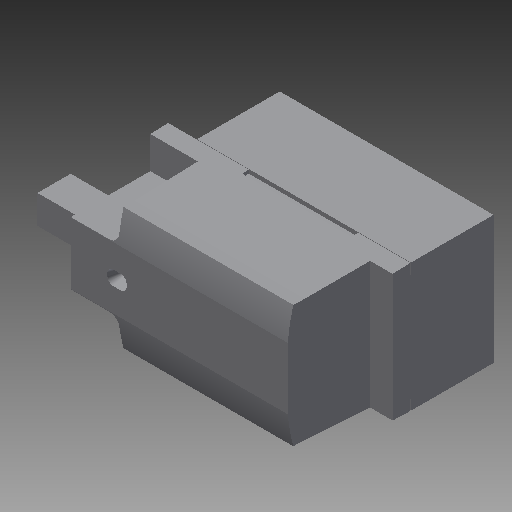
# Autodesk Inventor part: 100031_P3
Saved by Autodesk Inventor 2019.3 (Build 233278000, 278)
## iProperties
Category: PARTsolutions
Company: MOELLER
Created: 2018-12-14
Part Number: 100031_P3
Material: Generic
Catalog Web Link: www.cadenas.de
Description: NZM1-XS Part3-NZM1-XS
Vendor: MOELLER
Document SubType Name: Modeling
Designer: psadmin
Manufacturer: MOELLER
Mass: 356.118 g
Surface Area: 358.668 cm^2
Volume: 356.118 cm^3
Density: 1 g/cm^3
Appearance: PSOLRGB-192-192-192
PSOL_IDENT_0: {$CADENAS_DATA\23d-libs\moeller\circuit_breaker\parts\nzm1_xs_p3.prj},162 {VTYP=3D},{NB=100031_P3},{
PSOL_IDENT_1: LINA=100031},{NN=NZM1-XS Part3},{DATE=10.12.2018 21:07:48},{GEOMDATE=14.05.2018 10:43:05},{VERSION=}
PSOL_IDENT_2: ,{LINEID=60},{WBVAR=},{WBNUMERIC=}  {NB=100031_P3},{LINA=100031},{KT=DUMMY},{BMENB=100031},{EPLAN=}
NN: NZM1-XS Part3
NT: NZM1-XS
NB: 100031_P3
NBSYN: $BMENB._P3
LINA: 100031
BMENB: 100031
SUPPLIER: MOELLER
ARTICLENO: 100031_P3
BOMINFO: 100031
CREATOR: CADENAS GmbH
Title: 100031
Author: Cadenas PARTsolutions
Comments: NZM1-XS
Autodesk Inventor part; units mm, degrees
sketch "Sketch_2" plane through (0, 0, 0) normal (0, 1, 0) x (-1, 0, 0)
  line L0 (0, -26) -> (0, 15)
  line L1 (0, 15) -> (-91.3632, 15)
  line L2 (-91.3632, 15) -> (-92.533, -18.5)
  line L3 (-92.533, -18.5) -> (-102, -18.5)
  line L4 (-102, -18.5) -> (-102, -61)
  line L5 (-102, -61) -> (-12, -61)
  line L6 (-12, -61) -> (-12, -26)
  line L7 (-12, -26) -> (0, -26)
  constraints: 16 end point
extrude "Extrusion1" add sketch "Sketch_2" along normal mid plane 54
sketch "Sketch_3" plane through (0, 0, 0) normal (1, 0, 0) x (0, 1, 0)
  line L0 (-30, 19) -> (-30, -26)
  line L1 (-30, -26) -> (-27, -26)
  line L2 (-27, -26) -> (-25.75, 8.0894)
  line L3 (-25.75, 8.0894) -> (-25.75, 12.7365)
  arc A0 (-5.46, 15.3565) -> (-25.75, 12.7365) centre (-5.46, -64.5185) ccw
  line L4 (-5.46, 15.3565) -> (5.46, 15.3565)
  arc A1 (25.75, 12.7365) -> (5.46, 15.3565) centre (5.46, -64.5185) ccw
  line L5 (25.75, 12.7365) -> (25.75, 8.0894)
  line L6 (25.75, 8.0894) -> (27, -26)
  line L7 (27, -26) -> (30, -26)
  line L8 (30, -26) -> (30, 19)
  line L9 (30, 19) -> (-30, 19)
  constraints: 20 end point, 4 point on circle, 2 centre point
extrude "Extrusion2" cut sketch "Sketch_3" along normal blind 102
sketch "Sketch_4" plane through (0, 0, 0) normal (1, 0, 0) x (0, 1, 0)
  line L0 (22.5, -26) -> (22.5, -26.2)
  line L1 (22.5, -26.2) -> (27, -26.2)
  line L2 (27, -26.2) -> (27, -26)
  line L3 (27, -26) -> (22.5, -26)
  constraints: 8 end point
extrude "Extrusion3" cut sketch "Sketch_4" along normal blind 102
sketch "Sketch_5" plane through (0, 0, 0) normal (1, 0, 0) x (0, 1, 0)
  line L0 (-22.5, -26) -> (-27, -26)
  line L1 (-27, -26) -> (-27, -26.2)
  line L2 (-27, -26.2) -> (-22.5, -26.2)
  line L3 (-22.5, -26.2) -> (-22.5, -26)
  constraints: 8 end point
extrude "Extrusion4" cut sketch "Sketch_5" along normal blind 102
sketch "Sketch_6" plane through (0, 27, 0) normal (0, 1, 0) x (1, 0, 0)
  line L0 (34, 23.2) -> (80, 23.2)
  line L1 (80, 23.2) -> (80, 26)
  line L2 (80, 26) -> (34, 26)
  line L3 (34, 26) -> (34, 23.2)
  constraints: 8 end point
extrude "Extrusion5" cut sketch "Sketch_6" against normal blind 1.5
sketch "Sketch_7" plane through (0, -27, 0) normal (0, 1, 0) x (1, 0, 0)
  line L0 (34, 23.2) -> (80, 23.2)
  line L1 (80, 23.2) -> (80, 26)
  line L2 (80, 26) -> (34, 26)
  line L3 (34, 26) -> (34, 23.2)
  constraints: 8 end point
extrude "Extrusion6" cut sketch "Sketch_7" along normal blind 1.5
sketch "Sketch_8" plane through (0, 0, -18.5) normal (0, 0, 1) x (1, 0, 0)
  line L0 (-10, -30) -> (20, -30)
  line L1 (20, -30) -> (20, -16.8)
  arc A0 (20, -16.8) -> (16.4, -13.2) centre (16.4, -16.8) ccw
  line L2 (16.4, -13.2) -> (-5, -13.2)
  line L3 (-5, -13.2) -> (-5, 13.2)
  line L4 (-5, 13.2) -> (16.4, 13.2)
  arc A1 (16.4, 13.2) -> (20, 16.8) centre (16.4, 16.8) ccw
  line L5 (20, 16.8) -> (20, 30)
  line L6 (20, 30) -> (-10, 30)
  line L7 (-10, 30) -> (-10, -30)
  constraints: 16 end point, 4 point on circle, 2 centre point
extrude "Extrusion7" cut sketch "Sketch_8" along normal blind 38.5
sketch "Sketch_9" plane through (0, 0, 0) normal (1, 0, 0) x (0, 1, 0)
  arc A0 (-2.5617, 4) -> (-4, 2.5617) centre (0, 0) ccw
  line L0 (-4, 2.5617) -> (-4, -2.5617)
  arc A1 (-4, -2.5617) -> (-2.5617, -4) centre (0, 0) ccw
  line L1 (-2.5617, -4) -> (2.5617, -4)
  arc A2 (2.5617, -4) -> (4, -2.5617) centre (0, 0) ccw
  line L2 (4, -2.5617) -> (4, 2.5617)
  arc A3 (4, 2.5617) -> (2.5617, 4) centre (0, 0) ccw
  line L3 (2.5617, 4) -> (-2.5617, 4)
  constraints: 8 end point, 8 point on circle, 4 centre point
extrude "Extrusion8" add sketch "Sketch_9" against normal blind 12.5
sketch "Sketch_10" plane through (-2, 0, 0) normal (1, 0, 0) x (0, 0, -1)
  line L0 (-7, -5.02) -> (-5.02, -7)
  line L1 (-5.02, -7) -> (7, -7)
  line L2 (7, -7) -> (7, 7)
  line L3 (7, 7) -> (-7, 7)
  line L4 (-7, 7) -> (-7, -5.02)
  line L5 (-4.2, -1.3009) -> (-4.2, -1.7397)
  line L6 (-4.2, -1.7397) -> (-1.7397, -4.2)
  line L7 (-1.7397, -4.2) -> (-1.3009, -4.2)
  line L8 (-1.3009, -4.2) -> (-1.1009, -4)
  line L9 (-1.1009, -4) -> (2.5617, -4)
  arc A0 (2.5617, -4) -> (4, -2.5617) centre (0, 0) ccw
  line L10 (4, -2.5617) -> (4, 2.5617)
  arc A1 (4, 2.5617) -> (2.5617, 4) centre (0, 0) ccw
  line L11 (2.5617, 4) -> (-2.5617, 4)
  arc A2 (-2.5617, 4) -> (-4, 2.5617) centre (0, 0) ccw
  line L12 (-4, 2.5617) -> (-4, -1.1009)
  line L13 (-4, -1.1009) -> (-4.2, -1.3009)
  constraints: 28 end point, 6 point on circle, 3 centre point
extrude "Extrusion9" add sketch "Sketch_10" against normal blind 20
sketch "Sketch_11" plane through (-22, 0, 0) normal (1, 0, 0) x (0, 0, -1)
  line L0 (-2.195, -7) -> (0, -11.7072)
  line L1 (0, -11.7072) -> (2.195, -7)
  line L2 (2.195, -7) -> (-2.195, -7)
  constraints: 6 end point
extrude "Extrusion10" add sketch "Sketch_11" along normal blind 3
sketch "Sketch_1" plane through (0, 0, 10) normal (0, 0, 1) x (1, 0, 0)
  line L0 (16.804, 0.696) -> (16.804, -0.696)
  arc A0 (16.804, -0.696) -> (17.804, -1.696) centre (17.804, -0.696) ccw
  line L1 (17.804, -1.696) -> (21.196, -1.696)
  arc A1 (21.196, -1.696) -> (22.196, -0.696) centre (21.196, -0.696) ccw
  line L2 (22.196, -0.696) -> (22.196, 0.696)
  arc A2 (22.196, 0.696) -> (21.196, 1.696) centre (21.196, 0.696) ccw
  line L3 (21.196, 1.696) -> (17.804, 1.696)
  arc A3 (17.804, 1.696) -> (16.804, 0.696) centre (17.804, 0.696) ccw
  constraints: 8 end point, 8 point on circle, 4 centre point
extrude "Extrusion11" cut sketch "Sketch_1" along normal blind 8 draft 15
ref_plane "P3_XY" through (-12.5, 0, 0) normal (1, 0, 0) x (0, 0, -1)
ref_plane "P3_YZ" through (-12.5, 0, 0) normal (0, 0, -1) x (0, 1, 0)
ref_plane "P3_ZX" through (-12.5, 0, 0) normal (0, 1, 0) x (1, 0, 0)
body "Solid1"
